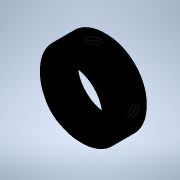
# Autodesk Inventor part: SCBRJ12-15_b
Saved by Autodesk Inventor 2021 (Build 250183000, 183)
## iProperties
Created: 2025-04-04
Part Number: SCBRJ12-15_b
Material: Generic
Catalog Web Link: www.cadenas.de
Description: SCBRJ, PSCBRJ, SSCBRJ, SCSRAJ, SCSRAWJ, SCBSJ, PSCBSJ, SSCBSJ_body-Set Collars - For Bearing Fixing - (For Space Saving) - Set Screw Compact Type
Vendor: MISUMI
Document SubType Name: Modeling
Designer: psAdmin
Manufacturer: MISUMI
Mass: 1.02882 g
Surface Area: 10.1631 cm^2
Volume: 1.02882 cm^3
Density: 1 g/cm^3
Appearance: PSOLRGB-0-0-0
Category: PARTsolutions
Company: MISUMI
Title: SCBRJ12-15
Author: Cadenas PARTsolutions
Comments: Set Collars - For Bearing Fixing - (For Space Saving) - Set Screw Compact Type
PSOL_IDENT_0: {$CADENAS_DATA/23d-libs/misumi/metric/03_set_collars/scbrj/scbrj_b.prj},238 {VTYP=3D},{NB=SCBRJ12-15
PSOL_IDENT_1: _b},{LINA=SCBRJ12-15},{NN=SCBRJ, PSCBRJ, SSCBRJ, SCSRAJ, SCSRAWJ, SCBSJ, PSCBSJ, SSCBSJ_body},{DATE=
PSOL_IDENT_2: 02.11.2021 00:56:13},{GEOMDATE=19.10.2021 09:28:48},{VERSION=},{LINEID=70},{WBVAR=TS,MAT,ST,DSS},{WB
PSOL_IDENT_3: NUMERIC=DSS}  {NB=SCBRJ12-15_b},{LINA=SCBRJ12-15},{KT=DUMMY},{PN=SCBRJ12-15},{D=12},{TYPE=SCBRJ},{TS=
PSOL_IDENT_4: SN},{MAT=1045},{MATA='1045','1045 Carbon Steel','304','SUS304 Equivalent','2017','2017 Aluminum Allo
PSOL_IDENT_5: y'},{ST=Black Oxide},{AC=Set Screws 2 Pcs.},{DSS=15},{DS1=15,16,18},{AB=6701ZZ(18)-6801ZZ(21)},{B11=
PSOL_IDENT_6: 7.5},{B12=10},{D1=19},{M=M4x3},{THMD=4},{THDMIN=3.242},{BB=6},{ST0='Black Oxide','Black Oxide','Elec
PSOL_IDENT_7: troless Nickel Plating','Electroless Nickel Plating'},{C=0.5},{L=3},{TS1='SN','Short Nose','LN','Lon
PSOL_IDENT_8: g Nose'},{COLOR=0.00,0.00,0.00,0.00},{B=7.5},{B1=0},{LTHREAD=3}
NB: SCBRJ12-15_b
NN: SCBRJ, PSCBRJ, SSCBRJ, SCSRAJ, SCSRAWJ, SCBSJ, PSCBSJ, SSCBSJ_body
NT: Set Collars - For Bearing Fixing - (For Space Saving) - Set Screw Compact Type
NBSYN: $PN._b
LINA: SCBRJ12-15
CATALOG: Misumi
PN: SCBRJ12-15
D: 12
TS: Short Nose
MAT: 1045 Carbon Steel
ST: Black Oxide
DSS: 15
D1: 19
M: M4x3
BB: 6
C: 0.5
L: 3
B: 7.5
B1: 0
SUPPLIER: MISUMI
ARTICLENO: SCBRJ12-15_b
BOMINFO: SCBRJ12-15
CREATOR: CADENAS GmbH
Autodesk Inventor part; units mm, degrees
sketch "Sketch_1" plane through (0, 0, 0) normal (0, 1, 0) x (-1, 0, 0)
  line L0 (0, 4.5) -> (0, -3)
  line L1 (-6, 4) -> (-6.5, 4.5)
  line L2 (-6.5, 4.5) -> (-7, 4.5)
  line L3 (-7, 4.5) -> (-7.5, 4)
  line L4 (-7.5, 4) -> (-7.5, 3)
  line L5 (-7.5, 3) -> (-9, 3)
  line L6 (-9, 3) -> (-9.5, 2.5)
  line L7 (-9.5, 2.5) -> (-9.5, -2.5)
  line L8 (-9.5, -2.5) -> (-9, -3)
  line L9 (-9, -3) -> (-6.5, -3)
  line L10 (-6.5, -3) -> (-6, -2.5)
  line L11 (-6, -2.5) -> (-6, 4)
  constraints: 24 end point
revolve "Revolution1" add sketch "Sketch_1" angle 360 about axis through (0, 0, 4.5) along (0, 0, -1)
sketch "Sketch_8" plane through (0, 0, 0) normal (0, 0, 1) x (1, 0, 0)
  line L0 (9.5, 0) -> (5, 0)
  line L1 (5, 0) -> (5, 1.621)
  line L2 (5, 1.621) -> (9.121, 1.621)
  line L3 (9.121, 1.621) -> (9.5, 2)
  line L4 (9.5, 2) -> (9.5, 0)
  line L5 (9.5, 0) -> (5, 0)
  constraints: 12 end point
revolve "Revolution2" cut sketch "Sketch_8" angle 360 about axis through (9.5, 0, 0) along (-1, 0, 0)
thread "Thread1" size "M4x0.7" class "6H" standard "ISO Metric profile" full length
sketch "Sketch_2" plane through (0, 0, 0) normal (0, 0, 1) x (1, 0, 0)
  line L0 (0, 9.5) -> (0, 5)
  line L1 (0, 5) -> (-1.621, 5)
  line L2 (-1.621, 5) -> (-1.621, 9.121)
  line L3 (-1.621, 9.121) -> (-2, 9.5)
  line L4 (-2, 9.5) -> (0, 9.5)
  line L5 (0, 9.5) -> (0, 5)
  constraints: 12 end point
revolve "Revolution3" cut sketch "Sketch_2" angle 360 about axis through (0, 9.5, 0) along (0, -1, 0)
thread "Thread2" size "M4x0.7" class "6H" standard "ISO Metric profile" full length
ref_plane "body_set_h_XY" through (0, 9.5, 0) normal (0, 1, 0) x (1, 0, 0)
ref_plane "body_set_h_YZ" through (0, 9.5, 0) normal (1, 0, 0) x (0, 0, -1)
ref_plane "body_set_h_ZX" through (0, 9.5, 0) normal (0, 0, -1) x (0, 1, 0)
ref_plane "body_set_v_XY" through (9.5, 0, 0) normal (1, 0, 0) x (0, 0, -1)
ref_plane "body_set_v_YZ" through (9.5, 0, 0) normal (0, 0, -1) x (0, 1, 0)
ref_plane "body_set_v_ZX" through (9.5, 0, 0) normal (0, 1, 0) x (1, 0, 0)
body "Solid1"
